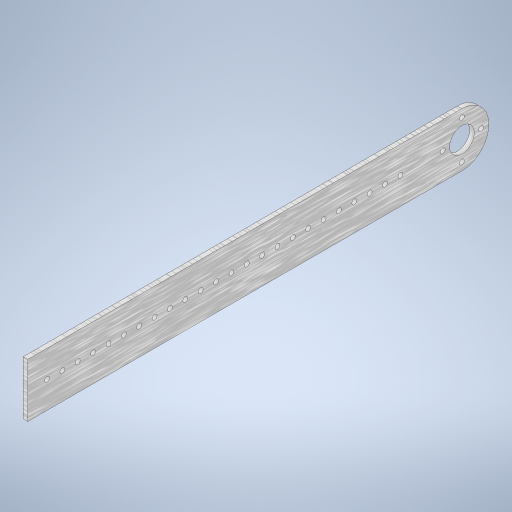
# Autodesk Inventor part: shoulder1_bottom_plate
Saved by Autodesk Inventor 2024 (Build 280153000, 153)
## iProperties
Company: 細田研究室
Created: 2025-06-07
Part Number: shoulder1_bottom_plate
Material: アルミニウム 5052
Document SubType Name: Modeling
Designer: HosodaLab2
Density: 2.68 g/cm^3
Appearance: サテン - ブラシ仕上げ 重厚
Mass: 70.367 g
Surface Area: 200.69 cm^2
Volume: 26.0618 cm^3
Stock Number: 1
個数: 1
Author: HosodaLab2
Autodesk Inventor part; units mm, degrees
ref_plane "YZ Plane" through (0, 0, 0) normal (1, 0, 0) x (0, 1, 0)
ref_plane "XZ Plane" through (0, 0, 0) normal (0, 1, 0) x (-1, 0, 0)
ref_plane "XY Plane" through (0, 0, 0) normal (0, 0, 1) x (1, 0, 0)
sketch "スケッチ1" plane through (0, 0, 0) normal (0, 1, 0) x (-1, 0, 0)
  line L0 (0, 0) -> (-300, 0)
  line L1 (-300, 0) -> (-300, -35)
  line L2 (-300, -35) -> (0, -35)
  line L3 (0, -35) -> (0, 0)
  arc A0 (-17.5, -35) -> (-17.5, 0) centre (-17.5, -17.5) ccw
  point P0 (-17.5, -17.5)
  dimension "d0" = 300
  dimension "d1" = 35
  dimension "d2" = 17.5
  dimension "d3" = 17.5
  dimension "d43" = 17.5
  constraints: 8 end point, 2 parallel, 2 point on circle, 2 point on line, 2 tangent, 1 centre point, 1 horizontal, 1 perpendicular
  measures "d0" distance of L2.end L1.end
  measures "d1" distance of L1.end L0.end
  measures "d2" distance from line of L2 point (-17.5, -17.5)
  measures "d3" distance from line of point (-17.5, -17.5) L3
  measures "d43" distance from line of L3 A0.centre
extrude "押し出し1" add sketch "スケッチ1" along normal blind 3 contours A0 L2 L1 L0
sketch "スケッチ2" plane through (0, 3, 0) normal (0, 1, 0) x (1, 0, 0)
  arc A0 (17.5, 35) -> (17.5, 0) centre (17.5, 17.5) ccw projected
  line L0 (300, 35) -> (17.5, 35) projected
  point P0 (0, 0)
  point P1 (0, 17.5)
  constraints: 1 coincident, 1 point on circle
hole "穴1" at (17.5, 3, -17.5) direction (0, -1, 0) diameter 16 end through all
sketch "スケッチ3" plane through (0, 3, 0) normal (0, 1, 0) x (1, 0, 0)
  line L0 (300, 0) -> (300, 35) projected
  arc A0 (17.5, 35) -> (17.5, 0) centre (17.5, 17.5) ccw construction
  line L1 (17.5, 17.5) -> (300, 17.5) construction
  line L2 (300, 0) -> (300, 35) construction
  point P0 (0, 0)
  point P1 (57.5, 17.5)
  point P2 (67.5, 17.5)
  point P3 (77.5, 17.5)
  point P4 (87.5, 17.5)
  point P5 (97.5, 17.5)
  point P6 (107.5, 17.5)
  point P7 (117.5, 17.5)
  point P8 (127.5, 17.5)
  point P9 (137.5, 17.5)
  point P10 (147.5, 17.5)
  point P11 (157.5, 17.5)
  point P12 (167.5, 17.5)
  point P13 (177.5, 17.5)
  point P14 (187.5, 17.5)
  point P15 (197.5, 17.5)
  point P16 (207.5, 17.5)
  point P17 (217.5, 17.5)
  point P18 (227.5, 17.5)
  point P19 (237.5, 17.5)
  point P20 (247.5, 17.5)
  point P21 (257.5, 17.5)
  point P22 (267.5, 17.5)
  point P23 (277.5, 17.5)
  point P24 (287.5, 17.5)
  dimension "d108" = 40
  dimension "d111" = 10
  constraints: 2 end point, 1 horizontal, 1 midpoint, 1 perpendicular, 1 point on line, 23 other
  measures "d108" distance of point (57.5, 17.5) L1.start
  measures "d111" distance of point (57.5, 17.5) point (67.5, 17.5)
hole "穴7" at (57.5, 3, -17.5) at (67.5, 3, -17.5) at (77.5, 3, -17.5) at (87.5, 3, -17.5) at (97.5, 3, -17.5) at (107.5, 3, -17.5) at (117.5, 3, -17.5) at (127.5, 3, -17.5) at (137.5, 3, -17.5) at (147.5, 3, -17.5) at (157.5, 3, -17.5) at (167.5, 3, -17.5) at (177.5, 3, -17.5) at (187.5, 3, -17.5) at (197.5, 3, -17.5) at (207.5, 3, -17.5) at (217.5, 3, -17.5) at (227.5, 3, -17.5) at (237.5, 3, -17.5) at (247.5, 3, -17.5) at (257.5, 3, -17.5) at (267.5, 3, -17.5) at (277.5, 3, -17.5) at (287.5, 3, -17.5) direction (0, -1, 0) diameter 3.2 end through all
sketch "スケッチ10" plane through (0, 3, 0) normal (0, 1, 0) x (1, 0, 0)
  circle A0 centre (17.5, 17.5) radius 8 construction
  circle A1 centre (17.5, 17.5) radius 12.5 construction
  point P0 (0, 0)
  point P1 (17.5, 5)
  point P2 (30, 17.5)
  point P3 (17.5, 30)
  point P4 (5, 17.5)
  dimension "d123" = 25
  dimension "d126" = 360
  constraints: 1 coincident, 1 vertical alignment, 7 other
hole "穴8" at (17.5, 3, -5) at (30, 3, -17.5) at (17.5, 3, -30) at (5, 3, -17.5) direction (0, -1, 0) diameter 3.2 end through all
